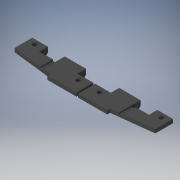
# Autodesk Inventor part: SoportePlaca_SPEL_Rev.3
Saved by Autodesk Inventor 2019.1 (Build 231200000, 200)
## iProperties
Created: 2018-09-11
Part Number: SoportePlaca_SPEL_Rev.3
Material: WindForm xt 2.0
Document SubType Name: Modeling
Designer: Elias
Density: 1.097 g/cm^3
Appearance: windform
Mass: 1.90579 g
Surface Area: 24.8341 cm^2
Volume: 1.73727 cm^3
Author: Elias
Autodesk Inventor part; units mm, degrees
sketch "Boceto1" plane through (0, 0, 0) normal (0, 1, 0) x (-1, 0, 0)
  line L0 (-40, -4.9) -> (40, -4.9)
  line L1 (40, -4.9) -> (40, 4.9)
  line L2 (40, 4.9) -> (-40, 4.9)
  line L3 (-40, 4.9) -> (-40, -4.9)
  line L4 (-40, -4.9) -> (40, 4.9) construction
  line L5 (40, -4.9) -> (-40, 4.9) construction
  point P0 (0, 0)
  dimension "d0" = 9.8
  dimension "d1" = 80
  constraints: 12 end point, 2 midpoint, 2 parallel, 1 horizontal, 1 perpendicular
  measures "d0" distance of L0.end L1.end
  measures "d1" distance of L0.start L0.end
extrude "Extrusión1" add sketch "Boceto1" along normal blind 2.2
sketch "Boceto4" plane through (0, 2.2, 0) normal (0, 1, 0) x (1, 0, 0)
  line L0 (40, 4.9) -> (-40, 4.9) projected
  line L1 (-40, -4.9) -> (40, -4.9) projected
  line L2 (23.5, 4.9) -> (21.5, 4.9)
  line L3 (21.5, 4.9) -> (21.5, -4.9)
  line L4 (21.5, -4.9) -> (23.5, -4.9)
  line L5 (23.5, -4.9) -> (23.5, 4.9)
  line L6 (40, -4.9) -> (40, 4.9) projected
  line L7 (0, 0) -> (0, 8.5747)
  line L8 (-23.5, 4.9) -> (-21.5, 4.9)
  line L9 (-21.5, 4.9) -> (-21.5, -4.9)
  line L10 (-21.5, -4.9) -> (-23.5, -4.9)
  line L11 (-23.5, -4.9) -> (-23.5, 4.9)
  point P0 (19.5, 4.9)
  dimension "d15" = 2
  dimension "d16" = 16.5
  constraints: 18 end point, 4 symmetric about line, 2 parallel, 2 point on line, 1 horizontal, 1 perpendicular, 1 vertical
  measures "d15" distance of L4.end L3.end
  measures "d16" distance between parallel lines of L6 L5
extrude "Extrusión4" cut sketch "Boceto4" against normal blind 0.8 contours L5 L1 L3 L0 | L9 L1 L11 L0
sketch "Boceto7" plane through (-40, 0, -4.9) normal (0, 0, -1) x (-1, 0, 0)
  line L0 (-80, 0) -> (0, 0) projected
  line L1 (-63.5, 2.2) -> (-80, 2.2) projected
  line L2 (-80, 0) -> (-73.5, 0)
  line L3 (-73.5, 0) -> (-73.5, 2.2)
  line L4 (-73.5, 2.2) -> (-80, 2.2)
  line L5 (-80, 2.2) -> (-80, 0)
  line L6 (-80, 0) -> (0, 0) projected
  line L7 (0, 2.2) -> (-16.5, 2.2) projected
  line L8 (0, 0) -> (-6.5, 0)
  line L9 (-6.5, 0) -> (-6.5, 2.2)
  line L10 (-6.5, 2.2) -> (0, 2.2)
  line L11 (0, 2.2) -> (0, 0)
  point P0 (-40, 0)
  point P1 (-59.5, 0)
  point P2 (-20.5, 0)
  dimension "d43" = 6.5
  dimension "d44" = 6.5
  constraints: 16 end point, 4 parallel, 2 horizontal, 2 perpendicular, 2 point on line
  measures "d43" distance of L4.end L3.end
  measures "d44" distance of L9.end L10.end
extrude "Extrusión7" add sketch "Boceto7" along normal blind 4.5
ref_plane "Plano de trabajo7" through (9.5, 0, -4.9) normal (0, 0, -1) x (-1, 0, 0)
sketch "Boceto8" plane through (9.5, 0, -4.9) normal (0, 0, -1) x (-1, 0, 0)
  line L0 (0, 2.2) -> (19, 2.2) projected
  line L1 (-24, 0) -> (43, 0) projected
  line L2 (-12, 2.2) -> (31, 2.2) projected
  line L3 (43, 0) -> (43, 2.2) projected
  line L4 (33, 2.2) -> (43, 2.2) projected
  line L5 (33, 2.2) -> (33, 1.4) projected
  line L6 (-12, 1.4) -> (-14, 1.4) projected
  line L7 (-24, 2.2) -> (-24, 0) projected
  line L8 (33, 1.4) -> (31, 1.4) projected
  line L9 (-14, 1.4) -> (-14, 2.2) projected
  line L10 (-24, 2.2) -> (-14, 2.2) projected
  line L11 (31, 1.4) -> (31, 2.2) projected
  line L12 (-12, 2.2) -> (-12, 1.4) projected
  point P0 (9.5, 0)
extrude "Extrusión8" cut sketch "Boceto8" against normal blind 0.3
sketch "Boceto11" plane through (0, 2.2, 0) normal (0, 1, 0) x (1, 0, 0)
  circle A0 centre (-36.1, 6.8) radius 1.1
  line L0 (-40, 9.4) -> (-33.5, 9.4) projected
  line L1 (-40, -4.9) -> (-40, 9.4) projected
  line L2 (0, 4.6) -> (0, 9.4)
  circle A1 centre (36.1, 6.8) radius 1.1
  point P0 (0, 0)
  dimension "d45" = 2.2
  dimension "d46" = 2.6
  dimension "d47" = 3.9
  constraints: 2 centre point, 2 end point, 1 symmetric about line, 1 vertical, 1 other
  measures "d45" diameter of A0
  measures "d46" distance from line of L0 A0.centre
  measures "d47" distance from line of L1 A0.centre
extrude "Extrusión11" cut sketch "Boceto11" against normal through all
sketch "Boceto14" plane through (0, 2.2, 0) normal (0, 1, 0) x (1, 0, 0)
  line L0 (-40, -4.9) -> (-40, 9.4) projected
  line L1 (-40, -4.9) -> (-40, -0.6)
  line L2 (-40, 9.4) -> (-33.5, 9.4) projected
  line L3 (0, 4.6) -> (0, 10.3532)
  line L4 (-40, -4.9) -> (-17, -4.9)
  line L5 (-17, -4.9) -> (-17, -3.3)
  line L6 (-17, -3.3) -> (-40, -0.6)
  line L7 (40, -4.9) -> (40, -0.6)
  line L8 (40, -4.9) -> (17, -4.9)
  line L9 (17, -4.9) -> (17, -3.3)
  line L10 (17, -3.3) -> (40, -0.6)
  point P0 (0, 0)
  point P1 (40, -4.9)
  dimension "d59" = 10
  dimension "d65" = 23
  dimension "d67" = 1.6
  constraints: 18 end point, 5 symmetric about line, 1 perpendicular, 1 point on line, 1 vertical
  measures "d59" distance from line of L2 L1.end
  measures "d65" distance of L0.start L4.end
  measures "d67" distance of L4.end L5.end
extrude "Extrusión14" cut sketch "Boceto14" against normal through all
ref_plane "Plano de trabajo5" through (0, 2.2, 0) normal (0, 1, 0) x (1, 0, 0)
sketch "Boceto15" plane through (0, 2.2, 0) normal (0, 1, 0) x (1, 0, 0)
  line L0 (0.5, -5.659) -> (-0.5, -5.659)
  line L1 (-0.5, -5.659) -> (-0.5, 5.659)
  line L2 (-0.5, 5.659) -> (0.5, 5.659)
  line L3 (0.5, 5.659) -> (0.5, -5.659)
  line L4 (0.5, -5.659) -> (-0.5, 5.659) construction
  line L5 (-0.5, -5.659) -> (0.5, 5.659) construction
  dimension "d69" = 1
  constraints: 12 end point, 2 parallel, 1 horizontal, 1 perpendicular
  measures "d69" distance of L1.end L2.end
extrude "Extrusión15" cut sketch "Boceto15" against normal through all
sketch "Boceto16" plane through (0, 2.2, 0) normal (0, 1, 0) x (1, 0, 0)
  circle A0 centre (-6, 1.6) radius 1.1
  line L0 (0, 0) -> (0, 8.3303)
  circle A1 centre (6, 1.6) radius 1.1
  line L1 (-0.5, 4.6) -> (-21.5, 4.6) projected
  line L2 (-0.5, -4.9) -> (-0.5, 4.6) projected
  dimension "d78" = 2.2
  dimension "d99" = 3
  dimension "d100" = 5.5
  constraints: 2 centre point, 2 end point, 1 symmetric about line, 1 vertical, 1 other
  measures "d78" diameter of A0
  measures "d99" distance from line of L1 A0.centre
  measures "d100" distance from line of L2 A0.centre
extrude "Extrusión16" cut sketch "Boceto16" against normal through all
sketch "Boceto17" plane through (0, 0, 0) normal (0, -1, 0) x (1, 0, 0)
  circle A0 centre (-6, -1.6) radius 1.1 projected
  line L0 (-17, 4.9) -> (-0.5, 4.9) projected
  line L1 (-17, 4.9) -> (-17, 3.3) projected
  line L2 (-17, 3.3) -> (-40, 0.6) projected
  line L3 (-40, 0.6) -> (-40, -9.4) projected
  line L4 (-33.5, -9.4) -> (-40, -9.4) projected
  circle A1 centre (-36.1, -6.8) radius 1.1 projected
  circle A2 centre (6, -1.6) radius 1.1 projected
  circle A3 centre (36.1, -6.8) radius 1.1 projected
  line L5 (40, -9.4) -> (33.5, -9.4) projected
  line L6 (40, 0.6) -> (40, -9.4) projected
  line L7 (40, 0.6) -> (17, 3.3) projected
  line L8 (17, 3.3) -> (17, 4.9) projected
  line L9 (0.5, 4.9) -> (17, 4.9) projected
  line L10 (-17, 3.3) -> (-40, 0.6) projected
  line L11 (-40, 0.6) -> (-40, -9.4) projected
  line L12 (-33.5, -9.4) -> (-40, -9.4) projected
  line L13 (-17, 4.9) -> (-17, 3.3) projected
  line L14 (40, -9.4) -> (33.5, -9.4) projected
  line L15 (40, 0.6) -> (40, -9.4) projected
  line L16 (40, 0.6) -> (17, 3.3) projected
  line L17 (17, 3.3) -> (17, 4.9) projected
  line L18 (-33.5, -9.4) -> (-33.5, -4.6) projected
  line L19 (33.5, -4.6) -> (33.5, -9.4) projected
  line L20 (-33.5, -9.4) -> (-33.5, -4.6) projected
  line L21 (33.5, -4.6) -> (33.5, -9.4) projected
  line L22 (0.5, 4.9) -> (0.5, -4.6) projected
  line L23 (-0.5, -4.6) -> (-0.5, 4.9) projected
  line L24 (-17, 4.9) -> (-0.5, 4.9) projected
  line L25 (0.5, 4.9) -> (0.5, -4.6) projected
  line L26 (0.5, 4.9) -> (17, 4.9) projected
  line L27 (-0.5, -4.6) -> (-0.5, 4.9) projected
  line L28 (0.5, -4.6) -> (33.5, -4.6) projected
  line L29 (-33.5, -4.6) -> (-0.5, -4.6) projected
  line L30 (0.5, -4.6) -> (33.5, -4.6) projected
  line L31 (-33.5, -4.6) -> (-0.5, -4.6) projected
  point P0 (0, 0)
extrude "Extrusión17" cut sketch "Boceto17" against normal blind 0.2
sketch "Boceto18" plane through (-33.5, 2.2, -4.9) normal (1, 0, 0) x (0, 0, -1)
  circle A0 centre (2.2, -2) radius 1.1
  line L0 (4.5, 0) -> (4.5, -2) projected
  line L1 (-0.3, 0) -> (4.5, 0) projected
  line L2 (-0.3, 0) -> (-0.3, -2) projected
  line L3 (4.5, 0) -> (-0.3, 0)
  line L4 (-0.3, 0) -> (-0.3, -2.4893)
  line L5 (1.2055, -4.2) -> (3.14, -4.2)
  line L6 (4.5, -2.7769) -> (4.5, 0)
  line L7 (4.5, -2.7769) -> (3.14, -4.2)
  line L8 (1.2055, -4.2) -> (-0.3, -2.4893)
  dimension "d89" = 2.2
  dimension "d90" = 1.1
  dimension "d91" = 2
  constraints: 12 end point, 2 parallel, 1 centre point, 1 horizontal, 1 perpendicular
  measures "d89" diameter of A0
  measures "d90" distance edge to line of A0 L5
  measures "d91" distance from line of A0.centre L1
extrude "Extrusión18" add sketch "Boceto18" along normal blind 2.3
sketch "Boceto20" plane through (-33.5, 2.2, -4.9) normal (-1, 0, 0) x (0, 0, 1)
  circle A0 centre (-2.2, -2) radius 1.1 projected
  point P0 (4.9, -2.2)
extrude "Extrusión19" add sketch "Boceto20" against normal blind 1.3
mirror "Simetría1" about plane through (0, 0, 0) normal (1, 0, 0) of "Extrusión19", "Extrusión18"
ref_plane "Plano de trabajo8" through (-9.5, 2.2, -9.4) normal (-1, 0, 0) x (0, 0, 1)
sketch "Boceto21" plane through (-9.5, 2.2, -9.4) normal (-1, 0, 0) x (0, 0, 1)
  circle A0 centre (2.3, -2) radius 1.1 projected
  line L0 (0, 0) -> (4.8, 0) projected
  line L1 (0, -2.7769) -> (0, 0) projected
  line L2 (1.36, -4.2) -> (0, -2.7769) projected
  line L3 (3.2945, -4.2) -> (1.36, -4.2) projected
  line L4 (4.8, -2.4893) -> (3.2945, -4.2) projected
  line L5 (4.8, -2) -> (4.8, -2.4893) projected
  line L6 (4.8, 0) -> (4.8, -2) projected
  point P0 (9.4, -2.2)
extrude "Extrusión20" add sketch "Boceto21" along normal blind 12
mirror "Simetría2" about plane through (0, 0, 0) normal (1, 0, 0) of "Extrusión20"
sketch "Boceto23" plane through (0, 0.2, 0) normal (0, -1, 0) x (1, 0, 0)
  line L0 (-23.5, 2.537) -> (-21.5, 2.7717) projected
  line L1 (-21.5, -4.6) -> (-21.5, 2.7717) projected
  line L2 (-21.5, -4.6) -> (-23.5, -4.6) projected
  line L3 (-23.5, 2.537) -> (-23.5, -4.6) projected
  line L4 (-23.5, -4.6) -> (-31.2, -4.6) projected
  line L5 (-24.5, -4.6) -> (-24.5, -1.6)
  line L6 (-24.5, -1.6) -> (-20.5, -1.6)
  line L7 (-20.5, -1.6) -> (-20.5, -4.6)
  line L8 (-20.5, -4.6) -> (-24.5, -4.6)
  line L9 (0, 0) -> (0, 8.701)
  line L10 (21.5, -4.6) -> (23.5, -4.6)
  line L11 (24.5, -4.6) -> (24.5, -1.6)
  line L12 (24.5, -1.6) -> (20.5, -1.6)
  line L13 (20.5, -1.6) -> (20.5, -4.6)
  line L14 (20.5, -4.6) -> (24.5, -4.6)
  dimension "d101" = 1
  dimension "d102" = 1
  dimension "d103" = 3
  constraints: 20 end point, 6 symmetric about line, 3 perpendicular, 2 vertical, 1 point on line
  measures "d101" distance between parallel lines of L5 L3
  measures "d102" distance between parallel lines of L1 L7
  measures "d103" distance of L6.end L7.end
extrude "Extrusión22" add sketch "Boceto23" along normal blind 0.4 contours L6 L1 L2 L3 | L3 L4 L5 L6 | L6 L7 L8 L1 | L14 L13 L12 L11 L10
chamfer "Chaflán3" distance 0.4 angle 45 1 edges at (20.5, 0.2, -3.1)
chamfer "Chaflán4" distance 0.4 angle 45 1 edges at (24.5, 0.2, -3.1)
chamfer "Chaflán5" distance 0.4 angle 45 2 edges at (-20.5, 0.2, -3.1) (-24.5, 0.2, -3.1)
